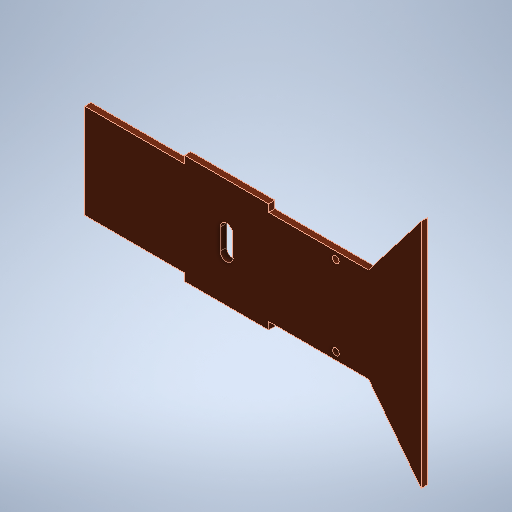
# Autodesk Inventor part: Path
Saved by Autodesk Inventor 2025.4 (Build 294407000, 407)
## iProperties
Created: 2026-04-06
Part Number: Path
Material: Generic
Document SubType Name: Sheet Metal
Designer: lenovo
Density: 1 g/cm^3
Sheet Metal Rule: Default_mm
Appearance: Default(1)
Author: lenovo
Autodesk Inventor part; units mm, degrees
ref_plane "YZ Plane" through (0, 0, 0) normal (1, 0, 0) x (0, 1, 0)
ref_plane "XZ Plane" through (0, 0, 0) normal (0, 1, 0) x (-1, 0, 0)
ref_plane "XY Plane" through (0, 0, 0) normal (0, 0, 1) x (1, 0, 0)
sketch "Sketch1" plane through (0, 0, 0) normal (0, 0, 1) x (1, 0, 0)
  line L0 (-67.5, -22.5) -> (67.5, -22.5)
  line L1 (67.5, -22.5) -> (67.5, 22.5)
  line L2 (67.5, 22.5) -> (-67.5, 22.5)
  line L3 (-67.5, 22.5) -> (-67.5, -22.5)
  line L4 (-67.5, -22.5) -> (67.5, 22.5) construction
  line L5 (67.5, -22.5) -> (-67.5, 22.5) construction
  line L6 (0, -5) -> (0, 5) construction
  line L7 (-3, -5) -> (-3, 5)
  line L8 (3, 5) -> (3, -5)
  arc A0 (-3, -5) -> (3, -5) centre (0, -5) ccw
  arc A1 (3, 5) -> (-3, 5) centre (0, 5) ccw
  line L9 (0, 0) -> (67.5, 0)
  circle A2 centre (52, 19) radius 1.6
  line L10 (-20, 26) -> (20, 26)
  line L11 (20, 26) -> (20, 22.5)
  line L12 (20, 22.5) -> (-20, 22.5)
  line L13 (-20, 22.5) -> (-20, 26)
  line L14 (-20, 26) -> (20, 22.5) construction
  line L15 (20, 26) -> (-20, 22.5) construction
  line L16 (-20, -26) -> (20, -26)
  line L17 (20, -26) -> (20, -22.5)
  line L18 (20, -22.5) -> (-20, -22.5)
  line L19 (-20, -22.5) -> (-20, -26)
  line L20 (-20, -26) -> (20, -22.5) construction
  line L21 (20, -26) -> (-20, -22.5) construction
  circle A3 centre (52, -19) radius 1.6
  point P0 (0, -8)
  point P1 (0, 8)
  point P2 (0, 24.25)
  point P3 (0, 22.5)
  point P4 (0, 22.5)
  point P5 (0, -24.25)
  point P6 (0, -22.5)
  point P7 (0, -22.5)
  dimension "d0" = 135
  dimension "d1" = 45
  dimension "d13" = 16
  dimension "d14" = 3
  dimension "d15" = 3.2
  dimension "d16" = 55
  dimension "d17" = 38
  dimension "d18" = 40
  dimension "d19" = 3.5
  measures "d0" distance of L1.end L2.end
  measures "d1" distance of L0.end L1.end
  measures "d13" distance of point (0, -8) point (0, 8)
  measures "d14" radius of A0
  measures "d15" diameter of A2
  measures "d16" distance from line of A2.centre L7
  measures "d17" diameter of A2.centre L9
  measures "d18" distance of L10.start L10.end
  measures "d19" distance of L10.end L11.end
sketch "Sketch2" plane through (0, 0, 1.5) normal (0, 0, 1) x (1, 0, 0)
  line L0 (67.5, -22.5) -> (67.5, 22.5)
  line L1 (67.5, -22.5) -> (92.5, -55)
  line L2 (67.5, 0) -> (0, 0)
  line L3 (67.5, 22.5) -> (92.5, 55)
  line L4 (92.5, 55) -> (92.5, -55)
  dimension "d20" = 25
  dimension "d21" = 110
  measures "d20" horizontal distance of L0.start L1.end
  measures "d21" distance of L3.end L1.end
extrude "Plate1" add sketch "Sketch1" along normal mid plane 3
sheet face with bend "Face2" sketch "Sketch2" thickness 3 toward (0, 0, -1) bend radius 3
bend "Bend1"
equation "\"d9\" = Thickness"
equation "\"d22\" = BendRadius"
equation "\"d23\" = BendReliefWidth"
equation "\"d25\" = MinimumRemnant"
equation "\"d24\" = BendReliefDepth"
equation "\"d26\" = TransitionRadius"
equation "\"BendRadius\" = Thickness"
equation "\"BendReliefWidth\" = Thickness"
equation "\"BendReliefDepth\" = 0.5 * Thickness"
equation "\"CornerReliefSize\" = 4 * Thickness"
equation "\"MinimumRemnant\" = 2 * Thickness"
equation "\"TransitionRadius\" = BendRadius"
equation "\"JacobiRadiusSize\" = BendRadius"
equation "\"GapSize\" = Thickness"
equation "\"Thickness\" = 3"
body "Solid1"
